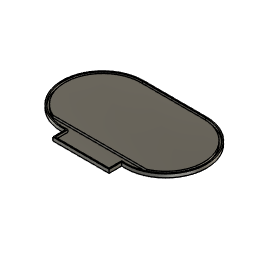
Wall Lamp Cover v10 (Autodesk Fusion 360 design; units mm, degrees)
Autodesk Fusion 360 part; units mm, degrees
sketch "Schizzo1" plane through (0, 0, 0) normal (0, 0, 1) x (1, 0, 0)
  line L0 (-52.948, 133.3465) -> (-52.948, -56.6535) construction
  line L1 (-107.948, 38.3465) -> (2.052, 38.3465) construction
  circle A0 centre (-107.948, 38.3465) radius 69.2
  circle A1 centre (-107.948, 38.3465) radius 71.2
  line L2 (2.052, 38.3465) -> (-107.948, 38.3465) construction
  circle A2 centre (2.052, 38.3465) radius 69.2
  circle A3 centre (2.052, 38.3465) radius 71.2
  line L3 (-107.948, 109.5465) -> (-107.948, -32.8535) construction
  line L4 (2.052, 109.5465) -> (2.052, -32.8535) construction
  line L5 (-107.948, 109.5465) -> (2.052, 109.5465)
  line L6 (-107.948, 107.5465) -> (2.052, 107.5465)
  line L7 (-5.948, -54.6535) -> (-99.948, -54.6535)
  line L8 (-99.948, -54.6535) -> (-99.948, -21.6535)
  line L9 (-99.948, -21.6535) -> (-5.948, -21.6535)
  line L10 (-5.948, -21.6535) -> (-5.948, -54.6535)
  line L11 (-5.948, -54.6535) -> (-99.948, -21.6535) construction
  line L12 (-99.948, -54.6535) -> (-5.948, -21.6535) construction
  line L13 (-3.948, -56.6535) -> (-101.948, -56.6535)
  line L14 (-101.948, -56.6535) -> (-101.948, -19.6535)
  line L15 (-101.948, -19.6535) -> (-3.948, -19.6535)
  line L16 (-3.948, -19.6535) -> (-3.948, -56.6535)
  line L17 (-3.948, -56.6535) -> (-101.948, -19.6535) construction
  line L18 (-101.948, -56.6535) -> (-3.948, -19.6535) construction
  line L19 (-101.948, -52.6535) -> (-3.948, -52.6535)
  line L20 (-99.948, -54.6535) -> (-101.948, -54.6535)
  line L21 (-5.948, -54.6535) -> (-3.948, -54.6535)
  circle A4 centre (-107.948, 38.3465) radius 65.8
  circle A5 centre (2.052, 38.3465) radius 65.8
  line L22 (-107.948, 104.1465) -> (2.052, 104.1465)
  line L23 (-101.948, -19.6535) -> (-149.245, -19.6535)
  line L24 (-3.948, -19.6535) -> (43.3489, -19.6535)
  line L25 (-99.948, -21.6535) -> (-146.2813, -21.6535)
  line L26 (-5.948, -21.6535) -> (40.3852, -21.6535)
  point P0 (-52.948, 38.3465)
  point P1 (-52.948, -38.1535)
  point P2 (-52.948, -38.1535)
  dimension "d1" = 138.4
  dimension "d2" = 142.4
  dimension "d3" = 110
  dimension "d4" = 94
  dimension "d5" = 33
  dimension "d6" = 60
  dimension "d7" = 37
  dimension "d8" = 98
  dimension "d10" = 2
  dimension "d18" = 131.6
  constraint vertical L0
  constraint perpendicular L0 L1
  constraint coincident L1.start A0.centre
  constraint concentric A0 A1
  constraint coincident L1 P0
  constraint coincident L0 P0
  constraint midpoint L0 L1
  constraint symmetric L0 L1.start L1.end
  constraint symmetric L0 L1.end L1.start
  constraint symmetric L0 A0 A2
  constraint symmetric L0 A1 A3
  constraint coincident A1 L3.start
  constraint coincident A1 L3.end
  constraint perpendicular L2 L3
  constraint coincident A3 L4.start
  constraint coincident A3 L4.end
  constraint perpendicular L2 L4
  constraint coincident A0 L6.start
  constraint coincident L3 L6.start
  constraint coincident L4 L6.end
  constraint coincident A2 L6.end
  constraint horizontal L7
  constraint perpendicular L7 L8
  constraint parallel L7 L9
  constraint parallel L8 L10
  constraint coincident L11 P2
  constraint coincident L12 P2
  constraint coincident L0 P2
  constraint horizontal L13
  constraint perpendicular L13 L14
  constraint parallel L13 L15
  constraint parallel L14 L16
  constraint coincident L17 P2
  constraint coincident L18 P2
  constraint coincident P2 P1
  constraint coincident L14 L19.start
  constraint coincident L16 L19.end
  constraint perpendicular L16 L19
  constraint coincident L14 L20.end
  constraint perpendicular L14 L20
  constraint coincident L16 L21.end
  constraint perpendicular L16 L21
  constraint coincident L1.start L3
  constraint coincident L1.end L4
  constraint coincident L0.end L13
  constraint concentric A1 A4
  constraint symmetric L0 A4 A5
  constraint coincident L3 L22.start
  constraint coincident A4 L22.start
  constraint coincident L4 L22.end
  constraint coincident A5 L22.end
  constraint coincident A1 L23.end
  constraint perpendicular L14 L23
  constraint coincident A3 L24.end
  constraint perpendicular L16 L24
  constraint coincident A1 L25.end
  constraint perpendicular L14 L25
  constraint coincident A3 L26.end
  constraint perpendicular L10 L26
  measures "d1" diameter of A0
  measures "d2" diameter of A1
  measures "d3" distance of L1.end L1.start
  measures "d4" distance of L8.end L9.end
  measures "d5" distance of L7.end L8.end
  measures "d6" distance of L2 L9
  measures "d7" distance of L13.end L14.end
  measures "d8" distance of L14 L16
  measures "d10" distance of L7 L19
  measures "d18" diameter of A4
extrude "Estrusione1" add sketch "Schizzo1" along normal blind 2 contours A0 A4 A5 | A0 A1 A5 | A0 A2 A4 A5 | A0 A1 A2 A5 | A0 A1 A2 A5 | A0 A2 A4 A5 | A0 A2 A3 A4 | A0 A1 A2 A3 | A1 L15 A5 L24 | A1 A2 A5 L22 | A2 A4 A5 | A4 A5 | A0 A1 A2 A3 | A0 A2 A3 A4 | A1 A2 L15 A5 | A0 A3 A4 L22 | A0 A1 A3 L22 | A1 A2 A3 L22 | A2 A3 A4 | A2 A5 L22 L24 | A0 A1 A3 L15 | A0 A3 L15 A4 | A1 A2 A3 L15 | A2 L9 L15 A5 | L9 L15 L16 A5 L26 | A0 A4 L22 L23 | A0 A1 L6 L22 | A1 A3 L22 | A3 L15 A4 L23 | A2 A3 L6 L22 | A0 A1 L9 L15 | A0 L9 L15 A4 | A1 A3 L15 | A2 A3 L9 L15 | L16 A5 L24 L26 | A2 L9 L10 A5 | L9 L10 A5 | A0 A1 L6 L23 | A1 A3 L6 L22 | A2 A3 L6 L24 | A2 A5 L24 L26 | A0 A1 L8 L9 | A0 L8 L9 A4 | L9 L14 L15 A4 L25 | A1 A3 L9 L15 | A2 A3 L9 L10 | L16 A5 L26 | L10 L16 A5 L26 | A2 L10 L16 A5 | A0 A4 L23 L25 | A0 A1 L23 L25 | A1 A3 L5 L6 | L14 A4 L23 L25 | A2 L16 A5 L26 | A2 A3 L24 L26 | A0 A1 L8 L14 | A0 L8 L14 A4 | L8 L9 A4 | A1 A3 L8 L9 L10 L19 | A2 A3 L10 L16 | A0 L14 A4 L25 | A0 A1 L14 L25 | L14 A4 L25 | A2 A3 L16 L26 | A1 L8 L14 L19 | L8 L14 A4 L25 | A3 L10 L16 L19 | L7 L8 L10 L19 | L8 L14 L19 L20 | L10 L16 L19 L21
extrude "Estrusione2" add sketch "Schizzo1" along normal blind 6 contours A0 A1 L6 L23 | A2 A3 L6 L24 | A0 A1 L23 L25 | A1 A3 L5 L6 | A2 A3 L24 L26 | A0 A1 L8 L14 | A2 A3 L10 L16 | A0 A1 L14 L25 | A2 A3 L16 L26 | A1 L8 L14 L19 | A3 L10 L16 L19 | L7 L8 L10 L19 | L8 L14 L19 L20 | L10 L16 L19 L21
extrude "Estrusione3" add sketch "Schizzo1" along normal blind 6 contours A0 A4 A5 | A0 A1 A5 | A0 A2 A4 A5 | A0 A1 A2 A5 | A0 A1 A2 A5 | A0 A2 A4 A5 | A0 A2 A3 A4 | A0 A1 A2 A3 | A1 L15 A5 L24 | A1 A2 A5 L22 | A2 A4 A5 | A4 A5 | A0 A1 A2 A3 | A0 A2 A3 A4 | A1 A2 L15 A5 | A0 A3 A4 L22 | A0 A1 A3 L22 | A1 A2 A3 L22 | A2 A3 A4 | A0 A1 A3 L15 | A0 A3 L15 A4 | A1 A2 A3 L15 | A2 L9 L15 A5 | L9 L15 L16 A5 L26 | A1 A3 L22 | A3 L15 A4 L23 | A0 A1 L9 L15 | A0 L9 L15 A4 | A1 A3 L15 | A2 A3 L9 L15 | L16 A5 L24 L26 | L9 L14 L15 A4 L25 | A1 A3 L9 L15 | L14 A4 L23 L25
equation "d1 = 138 mm + 0.40 mm"
equation "d2 = d1 + 4 mm"
equation "d5 = 29 mm + 4 mm"
equation "d7 = d5 + 4 mm"
equation "d8 = d4 + 4 mm"
equation "d18 = 132 mm - 0.4 mm"
